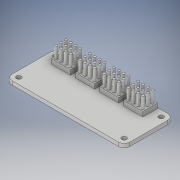
# Autodesk Inventor part: PCA9685
Saved by Autodesk Inventor 2018.2 (Build 222227000, 227)
## iProperties
Created: 2018-03-17
Part Number: PCA9685
Material: Generisch
Document SubType Name: Modeling
Designer: JochenAlt
Density: 1 g/cm^3
Appearance: Vorgabe
Author: JochenAlt
Autodesk Inventor part; units mm, degrees
ref_plane "YZ Plane" through (0, 0, 0) normal (1, 0, 0) x (0, 1, 0)
ref_plane "XZ Plane" through (0, 0, 0) normal (0, 1, 0) x (-1, 0, 0)
ref_plane "XY Plane" through (0, 0, 0) normal (0, 0, 1) x (1, 0, 0)
sketch "Skizze1" plane through (0, 0, 0) normal (0, 0, 1) x (1, 0, 0)
  line L0 (-28, 13) -> (28, 13)
  line L1 (31, 10) -> (31, -10)
  line L2 (28, -13) -> (-28, -13)
  line L3 (-31, -10) -> (-31, 10)
  circle A0 centre (-27.75, 9.75) radius 1.25
  circle A1 centre (27.75, 9.75) radius 1.25
  circle A2 centre (-27.75, -9.75) radius 1.25
  circle A3 centre (27.75, -9.75) radius 1.25
  line L4 (-27.75, 9.75) -> (27.75, 9.75) construction
  line L5 (27.75, 9.75) -> (27.75, -9.75) construction
  line L6 (27.75, -9.75) -> (-27.75, -9.75) construction
  line L7 (-27.75, -9.75) -> (-27.75, 9.75) construction
  line L8 (0, 19.0698) -> (0, -19.0698) construction
  line L9 (-44.2698, 0) -> (44.2698, 0) construction
  arc A4 (31, 10) -> (28, 13) centre (28, 10) ccw
  arc A5 (28, -13) -> (31, -10) centre (28, -10) ccw
  arc A6 (-28, 13) -> (-31, 10) centre (-28, 10) ccw
  arc A7 (-31, -10) -> (-28, -13) centre (-28, -10) ccw
  circle A8 centre (-24, 11.23) radius 0.6689
  circle A9 centre (-24, 8.69) radius 0.6689
  circle A10 centre (-24, 6.15) radius 0.6689
  line L10 (-24, 11.23) -> (-24, 6.15) construction
  line L11 (-21.46, 11.23) -> (-21.46, 6.15) construction
  circle A11 centre (-21.46, 11.23) radius 0.6689
  circle A12 centre (-21.46, 8.69) radius 0.6689
  circle A13 centre (-21.46, 6.15) radius 0.6689
  line L12 (-18.92, 11.23) -> (-18.92, 6.15) construction
  circle A14 centre (-18.92, 11.23) radius 0.6689
  circle A15 centre (-18.92, 8.69) radius 0.6689
  circle A16 centre (-18.92, 6.15) radius 0.6689
  line L13 (-16.38, 11.23) -> (-16.38, 6.15) construction
  circle A17 centre (-16.38, 11.23) radius 0.6689
  circle A18 centre (-16.38, 8.69) radius 0.6689
  circle A19 centre (-16.38, 6.15) radius 0.6689
  line L14 (-25.27, 12.5) -> (-15.11, 12.5)
  line L15 (-15.11, 12.5) -> (-15.11, 4.88)
  line L16 (-15.11, 4.88) -> (-25.27, 4.88)
  line L17 (-25.27, 4.88) -> (-25.27, 12.5)
  point P0 (0, 0)
  dimension "d0" = 62
  dimension "d1" = 26
  dimension "d2" = 2.5
  dimension "d3" = 55.5
  dimension "d4" = 19.5
  dimension "d5" = 3
  dimension "d8" = 2.54
  dimension "d9" = 2.54
  dimension "d12" = 2.54
  dimension "d17" = 1.27
  dimension "d18" = 1.27
  dimension "d19" = 1.27
  dimension "d20" = 1.27
  dimension "d28" = 7
  dimension "d29" = 0.5
  constraints: 32 end point, 20 centre point, 8 equal radius, 8 point on circle, 8 tangent, 6 parallel, 4 horizontal, 3 perpendicular, 2 coincident, 1 midpoint, 1 vertical, 25 other
  measures "d0" distance between parallel lines of L1 L3
  measures "d1" distance between parallel lines of L2 L0
  measures "d2" diameter of A1
  measures "d3" distance between parallel lines of L5 L7
  measures "d4" distance between parallel lines of L6 L4
  measures "d5" radius of A4
  measures "d8" distance of A9.centre L10.start
  measures "d9" distance of A9.centre L10.end
  measures "d12" distance of L10.start L11.start
  measures "d17" distance between parallel lines of L13 L15
  measures "d18" distance from line of L13.start L14
  measures "d19" distance from line of L16 L13.end
  measures "d20" distance between parallel lines of L17 L10
  measures "d28" distance between parallel lines of L10 L3
  measures "d29" distance between parallel lines of L0 L14
extrude "Extrusion1" add sketch "Skizze1" along normal blind 2 contours L0 A4 L1 A5 L2 A7 L3 A6 | A8 | A9 | A10 | A11 | A12 | A13 | A14 | A15 | A16 | A17 | A18 | A19 | L14 L15 L16 L17
extrude "Extrusion2" add sketch "Skizze1" along normal blind 4.5 contours L14 L15 L16 L17
extrude "Extrusion3" add sketch "Skizze1" along normal blind 10.5 contours A8 | A9 | A10 | A11 | A12 | A13 | A14 | A15 | A16 | A17 | A18 | A19
pattern_linear "Rechteckige Anordnung1" count 4 spacing 12.7 along (1, 0, 0) of "Extrusion2", "Extrusion3"
equation "\"d9\" = d8"
equation "\"d19\" = d18"
equation "\"d20\" = d17"
